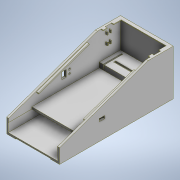
# Autodesk Inventor part: main
Saved by Autodesk Inventor 2021 (Build 250183000, 183)
## iProperties
Created: 2019-01-15
Part Number: main
Material: ABS 塑料(1)
Document SubType Name: Modeling
Designer: Guo Xin
Density: 1.06 g/cm^3
Appearance: 平滑 - 白色(1)
Author: Guo Xin
Autodesk Inventor part; units mm, degrees
note: some values were not read from the file. Chosen so that the rebuilt part matches the saved one: second side of "拉伸16".
ref_plane "YZ Plane" through (0, 0, 0) normal (1, 0, 0) x (0, 1, 0)
ref_plane "XZ Plane" through (0, 0, 0) normal (0, 1, 0) x (-1, 0, 0)
ref_plane "XY Plane" through (0, 0, 0) normal (0, 0, 1) x (1, 0, 0)
sketch "草图1" plane through (0, 0, 0) normal (0, 1, 0) x (-1, 0, 0)
  line L0 (0, 0) -> (80, 0)
  line L1 (80, 0) -> (80, -172)
  line L2 (80, -172) -> (0, -172)
  line L3 (0, -172) -> (0, 0)
  dimension "d0" = 172
  dimension "d1" = 80
  constraints: 8 end point, 2 parallel, 1 horizontal, 1 perpendicular
  measures "d0" distance between parallel lines of L2 L0
  measures "d1" distance between parallel lines of L3 L1
extrude "拉伸1" add sketch "草图1" along normal blind 70
sketch "草图2" plane through (-80, 0, 0) normal (0, 0, 1) x (1, 0, 0)
  line L0 (2.5, 16.5) -> (77.5, 16.5)
  line L1 (77.5, 16.5) -> (77.5, 3)
  line L2 (77.5, 3) -> (2.5, 3)
  line L3 (2.5, 3) -> (2.5, 16.5)
  line L4 (80, 0) -> (0, 0) projected
  line L5 (80, 0) -> (80, 70) projected
  line L6 (0, 0) -> (0, 70) projected
  dimension "d4" = 3
  dimension "d5" = 2.5
  dimension "d6" = 2.5
  dimension "d7" = 13.5
  dimension "d225" = 75
  constraints: 8 end point, 2 parallel, 1 horizontal, 1 perpendicular
  measures "d4" distance between parallel lines of L4 L2
  measures "d5" distance between parallel lines of L5 L1
  measures "d6" distance between parallel lines of L6 L3
  measures "d7" distance between parallel lines of L2 L0
  measures "d225" distance between parallel lines of L1 L3
extrude "拉伸2" cut sketch "草图2" against normal blind 170
sketch "草图3" plane through (0, 70, 0) normal (0, 1, 0) x (1, 0, 0)
  line L0 (-66.25, 151) -> (-13.75, 151)
  line L1 (-13.75, 151) -> (-13.75, 148)
  line L2 (-13.75, 148) -> (-66.25, 148)
  line L3 (-66.25, 148) -> (-66.25, 151)
  line L4 (0, 172) -> (-80, 172) projected
  line L5 (-80, 172) -> (-80, 0) projected
  line L6 (0, 0) -> (0, 172) projected
  dimension "d10" = 52.5
  dimension "d11" = 3
  dimension "d12" = 21
  dimension "d13" = 13.75
  dimension "d14" = 80
  constraints: 8 end point, 2 parallel, 1 horizontal, 1 perpendicular
  measures "d10" distance between parallel lines of L1 L3
  measures "d11" distance between parallel lines of L2 L0
  measures "d12" distance between parallel lines of L4 L0
  measures "d13" distance between parallel lines of L5 L3
  measures "d14" distance between parallel lines of L6 L5
extrude "拉伸3" cut sketch "草图3" against normal blind 45
sketch "草图4" plane through (0, 0, 0) normal (1, 0, 0) x (0, 0, -1)
  line L0 (137, 70) -> (0, 22)
  line L1 (172, 0) -> (172, 70) projected
  line L2 (172, 0) -> (0, 0) projected
  line L3 (0, 0) -> (0, 70) projected
  line L4 (0, 70) -> (172, 70) projected
  dimension "d17" = 35
  dimension "d18" = 22
  constraints: 2 end point, 2 point on line
  measures "d17" distance from line of L1 L0.start
  measures "d18" distance from line of L2 L0.end
extrude "拉伸4" cut sketch "草图4" against normal blind 80 contours L0 L3 L4
sketch "草图5" plane through (0, 70, 0) normal (0, 1, 0) x (1, 0, 0)
  line L0 (-77, 137) -> (-3, 137)
  line L1 (-3, 137) -> (-3, 0)
  line L2 (-3, 0) -> (-77, 0)
  line L3 (-77, 0) -> (-77, 137)
  line L4 (-80, 0) -> (-80, 137) projected
  line L5 (0, 137) -> (0, 0) projected
  line L6 (-80, 137) -> (0, 137) projected
  line L7 (0, 0) -> (-80, 0) projected
  point P0 (-76, 137)
  point P1 (-76, 0)
  dimension "d21" = 3
  dimension "d22" = 3
  constraints: 8 end point, 2 collinear, 2 parallel, 1 horizontal, 1 perpendicular
  measures "d21" distance between parallel lines of L4 L3
  measures "d22" distance between parallel lines of L5 L1
extrude "拉伸5" cut sketch "草图5" against normal blind 48 contours L0 L1 L2 L3
sketch "草图9" plane through (-77, 70, -137) normal (0, 0, 1) x (1, 0, 0)
  line L0 (3, -3) -> (71, -3)
  line L1 (71, -3) -> (71, -43)
  line L2 (71, -43) -> (3, -43)
  line L3 (3, -43) -> (3, -3)
  line L4 (0, 0) -> (74, 0) projected
  line L5 (0, -48) -> (0, 0) projected
  line L6 (74, 0) -> (74, -48) projected
  line L7 (2.5, -48) -> (71.5, -48) projected
  point P0 (77, -70)
  dimension "d34" = 3
  dimension "d35" = 3
  dimension "d36" = 3
  dimension "d226" = 40
  constraints: 8 end point, 2 parallel, 1 horizontal, 1 perpendicular
  measures "d34" distance between parallel lines of L4 L0
  measures "d35" distance between parallel lines of L5 L3
  measures "d36" distance between parallel lines of L6 L1
  measures "d226" distance between parallel lines of L2 L0
extrude "拉伸8" cut sketch "草图9" against normal blind 32
sketch "草图12" plane through (-74, 27, -137) normal (1, 0, 0) x (0, 0, -1)
  line L0 (11, 40) -> (14, 40)
  line L1 (14, 40) -> (14, 0)
  line L2 (14, 0) -> (11, 0)
  line L3 (11, 0) -> (11, 40)
  line L4 (11, 43) -> (11, 40) projected
  line L5 (14, 43) -> (14, 40) projected
  line L6 (11, 40) -> (14, 40) projected
  line L7 (0, 0) -> (32, 0) projected
  point P0 (-137, -27)
  point P1 (11, -2)
  point P2 (14, -2)
  dimension "d40" = 0
  dimension "d41" = 0
  constraints: 8 end point, 2 collinear, 2 parallel, 1 horizontal, 1 perpendicular
  measures "d40" distance between parallel lines of L4 L3
  measures "d41" distance between parallel lines of L5 L1
extrude "拉伸9" cut sketch "草图12" against normal blind 3 and the other way blind 71
sketch "草图15" plane through (-74, 27, -137) normal (1, 0, 0) x (0, 0, -1)
  line L0 (0, 40) -> (6.5, 40)
  line L1 (6.5, 40) -> (6.5, 0)
  line L2 (6.5, 0) -> (0, 0)
  line L3 (0, 0) -> (0, 40)
  line L4 (0, 0) -> (0, 40) projected
  line L5 (0, 0) -> (32, 0) projected
  line L6 (0, 40) -> (32, 40) projected
  line L7 (11, 0) -> (11, 40) projected
  point P0 (-137, -27)
  dimension "d44" = 4.5
  constraints: 8 end point, 3 collinear, 2 parallel, 1 horizontal, 1 perpendicular
  measures "d44" distance between parallel lines of L7 L1
extrude "拉伸10" cut sketch "草图15" against normal blind 3 and the other way blind 71 contours L0 L1 L2 L3
sketch "草图16" plane through (-74, 27, -169) normal (1, 0, 0) x (0, 0, -1)
  line L0 (-13.5, 40) -> (0, 40)
  line L1 (0, 40) -> (0, 0)
  line L2 (0, 0) -> (-13.5, 0)
  line L3 (-13.5, 0) -> (-13.5, 40)
  line L4 (-18, 0) -> (0, 0) projected
  line L5 (-18, 40) -> (0, 40) projected
  line L6 (-18, 40) -> (-18, 0) projected
  line L7 (0, 0) -> (0, 40) projected
  point P0 (-169, -27)
  dimension "d47" = 4.5
  constraints: 8 end point, 3 collinear, 2 parallel, 1 horizontal, 1 perpendicular
  measures "d47" distance between parallel lines of L6 L3
extrude "拉伸11" cut sketch "草图16" against normal blind 3 and the other way blind 71 contours L0 L1 L2 L3
sketch "草图17" plane through (-74, 27, -148) normal (1, 0, 0) x (0, 0, -1)
  line L0 (-0.75, 40) -> (3.75, 40)
  line L1 (3.75, 40) -> (3.75, 19)
  line L2 (3.75, 19) -> (-0.75, 19)
  line L3 (-0.75, 19) -> (-0.75, 40)
  line L4 (3, 40) -> (7.5, 40) projected
  line L5 (0, 0) -> (0, 40) projected
  line L6 (3, 0) -> (7.5, 0) projected
  point P0 (-148, -27)
  dimension "d50" = 0.75
  dimension "d51" = 4.5
  dimension "d52" = 19
  constraints: 8 end point, 2 parallel, 1 collinear, 1 horizontal, 1 perpendicular
  measures "d50" distance between parallel lines of L5 L3
  measures "d51" distance between parallel lines of L1 L3
  measures "d52" distance between parallel lines of L6 L2
extrude "拉伸12" cut sketch "草图17" against normal blind 3 and the other way blind 71
sketch "草图18" plane through (-74, 27, -143.5) normal (1, 0, 0) x (0, 0, -1)
  line L0 (0, 18) -> (12, 18)
  line L1 (12, 18) -> (12, 0)
  line L2 (12, 0) -> (0, 0)
  line L3 (0, 0) -> (0, 18)
  line L4 (0, 40) -> (0, 0) projected
  line L5 (12, 0) -> (12, 40) projected
  line L6 (7.5, 0) -> (12, 0) projected
  line L7 (8.25, 19) -> (3.75, 19) projected
  point P0 (-143.5, -27)
  point P1 (4.5, 19)
  dimension "d55" = 1
  constraints: 8 end point, 3 collinear, 2 parallel, 1 horizontal, 1 perpendicular
  measures "d55" distance between parallel lines of L0 L7
extrude "拉伸13" cut sketch "草图18" against normal blind 3 and the other way blind 71
sketch "草图19" plane through (-74, 46, -147.25) normal (1, 0, 0) x (0, 0, -1)
  line L0 (-3.75, 21) -> (-1, 21)
  line L1 (-1, 21) -> (-1, -1)
  line L2 (-1, -1) -> (-3.75, -1)
  line L3 (-3.75, -1) -> (-3.75, 21)
  line L4 (5.5, 21) -> (8.25, 21)
  line L5 (8.25, 21) -> (8.25, -1)
  line L6 (8.25, -1) -> (5.5, -1)
  line L7 (5.5, -1) -> (5.5, 21)
  line L8 (2.25, 24.0103) -> (2.25, -3.9452)
  line L9 (0, 0) -> (0, 21) projected
  line L10 (-3.75, 21) -> (0, 21) projected
  line L11 (-3.75, 21) -> (-3.75, -1) projected
  line L12 (-3.75, -1) -> (8.25, -1) projected
  point P0 (-147.25, -46)
  point P1 (0.75, -1)
  dimension "d58" = 2.25
  dimension "d59" = 2
  constraints: 18 end point, 4 parallel, 3 collinear, 2 horizontal, 2 perpendicular, 1 point on line, 1 vertical, 3 other
  measures "d58" distance between parallel lines of L8 L9
  measures "d59" diameter of L1 L9
extrude "拉伸14" cut sketch "草图19" against normal blind 3 and the other way blind 71
sketch "草图20" plane through (-74, 46, -147.25) normal (1, 0, 0) x (0, 0, -1)
  line L0 (-1, 13) -> (5.5, 13)
  line L1 (5.5, 13) -> (5.5, 3)
  line L2 (5.5, 3) -> (-1, 3)
  line L3 (-1, 3) -> (-1, 13)
  line L4 (-1, 21) -> (-1, -1) projected
  line L5 (5.5, -1) -> (5.5, 21) projected
  line L6 (-1, -1) -> (5.5, -1) projected
  line L7 (0.75, 21) -> (3.75, 21) projected
  line L8 (0, 13) -> (-1, 13)
  line L9 (0, 0) -> (0, 21) projected
  line L10 (-1, 21) -> (0, 21) projected
  point P0 (-147.25, -46)
  point P1 (0.75, -1)
  dimension "d62" = 4
  dimension "d63" = 8
  constraints: 10 end point, 3 collinear, 2 parallel, 1 horizontal, 1 perpendicular
  measures "d62" distance between parallel lines of L6 L2
  measures "d63" distance between parallel lines of L7 L0
extrude "拉伸15" cut sketch "草图20" against normal blind 3 and the other way blind 71 contours L0 L9 L2 L3 | L0 L1 L2 L9
sketch "草图21" plane through (0, 22, 0) normal (0, 1, 0) x (1, 0, 0)
  line L0 (-71.25, 165) -> (-69.5, 165)
  line L1 (-69.5, 165) -> (-69.5, 135)
  line L2 (-69.5, 135) -> (-71.25, 135)
  line L3 (-71.25, 135) -> (-71.25, 165)
  line L4 (-10.5, 165) -> (-8.75, 165)
  line L5 (-8.75, 165) -> (-8.75, 135)
  line L6 (-8.75, 135) -> (-10.5, 135)
  line L7 (-10.5, 135) -> (-10.5, 165)
  line L8 (-3, 135) -> (-77, 135) projected
  line L9 (-66.25, 148) -> (-66.25, 151) projected
  line L10 (-2.5, 170) -> (-77.5, 170) projected
  line L11 (-80, 0) -> (-80, 172) projected
  line L12 (-40, 178.7655) -> (-40, 86)
  point P0 (0, 0)
  dimension "d94" = 5
  dimension "d95" = 1.75
  dimension "d96" = 5
  dimension "d97" = 10.5
  dimension "d188" = 80
  constraints: 18 end point, 4 parallel, 2 horizontal, 2 perpendicular, 1 collinear, 1 point on line, 1 vertical, 3 other
  measures "d94" distance between parallel lines of L9 L3
  measures "d95" distance between parallel lines of L1 L3
  measures "d96" distance between parallel lines of L10 L0
  measures "d97" distance between parallel lines of L11 L1
  measures "d188" diameter of L11 L12
extrude "拉伸16" cut sketch "草图21" along normal blind 5
sketch "草图29" plane through (-74, 67, -146.25) normal (1, 0, 0) x (0, 0, -1)
  line L0 (0, 0) -> (6.5, 0)
  line L1 (6.5, 0) -> (6.5, -4)
  line L2 (6.5, -4) -> (0, -4)
  line L3 (0, -4) -> (0, 0)
  line L4 (0, 0) -> (1, 0) projected
  line L5 (0, 0) -> (0, -8) projected
  line L6 (6.5, -8) -> (6.5, 0) projected
  point P0 (-146.25, -67)
  dimension "d248" = 4
  constraints: 8 end point, 3 collinear, 2 parallel, 1 horizontal, 1 perpendicular
  measures "d248" distance between parallel lines of L2 L0
extrude "拉伸20" cut sketch "草图29" against normal blind 3 and the other way blind 65
sketch "草图30" plane through (-3, 27, -169) normal (-1, 0, 0) x (0, 0, 1)
  line L0 (32, 41.9404) -> (32, 39.8212)
  line L1 (32, 39.8212) -> (127.0364, 6.5238)
  line L2 (127.0364, 6.5238) -> (127.0364, 8.643)
  line L3 (127.0364, 8.643) -> (32, 41.9404)
  line L4 (32, 43) -> (32, 40) projected
  line L5 (32, 39.8212) -> (32.992, 42.6524)
  line L6 (32, 43) -> (169, -5) projected
  line L7 (127.0364, 8.643) -> (126.3751, 6.7555)
  line L8 (32, 39.8212) -> (126.3751, 6.7555)
  line L9 (126.3751, 6.7555) -> (126.7057, 7.6992)
  line L10 (126.7057, 7.6992) -> (32.3307, 40.7649)
  line L11 (32.3307, 40.7649) -> (32, 39.8212)
  point P0 (169, -27)
  point P1 (169, -5)
  point P2 (32, -5)
  point P3 (157.5833, 0)
  dimension "d144" = 1
  dimension "d145" = 2
  dimension "d146" = 100
  dimension "d147" = 2
  dimension "d148" = 1
  constraints: 20 end point, 3 collinear, 3 parallel, 3 perpendicular, 1 point on line, 1 vertical, 5 other
  measures "d145" distance between parallel lines of L1 L3
  measures "d146" distance between parallel lines of L7 L5
  measures "d147" distance between parallel lines of L3 L8
  measures "d148" distance between parallel lines of L1 L10
extrude "拉伸21" add sketch "草图30" along normal blind 74 contours L3 L5 L0 | L3 L7 L10 L5 | L5 L10 L7 L1
sketch "草图31" plane through (-77, 35.643, -41.9636) normal (0, 0.9437509, 0.3306573) x (1, 0, 0)
  line L0 (3, 101.0511) -> (71, 101.0511)
  line L1 (71, 101.0511) -> (71, 0)
  line L2 (71, 0) -> (3, 0)
  line L3 (3, 0) -> (3, 101.0511)
  line L4 (0, 101.0511) -> (74, 101.0511) projected
  line L5 (74, 0) -> (0, 0) projected
  line L6 (0, -44.1143) -> (0, 101.0511) projected
  line L7 (74, 101.0511) -> (74, -44.1143) projected
  point P0 (77, -51.3888)
  point P1 (4, 0)
  point P2 (0, -32.0172)
  point P3 (74, -32.0172)
  dimension "d151" = 3
  dimension "d152" = 3
  constraints: 8 end point, 2 collinear, 2 parallel, 1 horizontal, 1 perpendicular
  measures "d151" distance between parallel lines of L6 L3
  measures "d152" distance between parallel lines of L7 L1
extrude "拉伸22" cut sketch "草图31" against normal blind 2 contours L0 L1 L2 L3
sketch "草图36" plane through (0, 0, 0) normal (0, -1, 0) x (1, 0, 0)
  line L0 (-13.5, 0) -> (-66.5, 0)
  line L1 (-66.5, 0) -> (-66.5, -10)
  line L2 (-66.5, -10) -> (-13.5, -10)
  line L3 (-13.5, -10) -> (-13.5, 0)
  line L4 (-80, 0) -> (-80, -172) projected
  line L5 (0, -172) -> (0, 0) projected
  line L6 (0, 0) -> (-80, 0) projected
  dimension "d159" = 80
  dimension "d160" = 13.5
  dimension "d161" = 13.5
  dimension "d162" = 10
  constraints: 8 end point, 2 parallel, 1 collinear, 1 horizontal, 1 perpendicular
  measures "d159" distance between parallel lines of L4 L5
  measures "d160" distance between parallel lines of L3 L5
  measures "d161" distance between parallel lines of L4 L1
  measures "d162" distance between parallel lines of L0 L2
extrude "拉伸23" cut sketch "草图36" against normal blind 1
sketch "草图37" plane through (0, 1, 0) normal (0, -1, 0) x (1, 0, 0)
  line L0 (-13.5, 0) -> (-13.5, -10) projected
  line L1 (-66.5, -10) -> (-66.5, 0) projected
  line L2 (-13.5, -10) -> (-66.5, -10) projected
  point P0 (0, 0)
  point P1 (-21.5, -4)
  point P2 (-58.5, -4)
  dimension "d165" = 8
  dimension "d166" = 8
  dimension "d167" = 6
  dimension "d168" = 6
  measures "d165" distance from line of L0 point (-21.5, -4)
  measures "d166" distance from line of L1 point (-58.5, -4)
  measures "d167" distance from line of L2 point (-21.5, -4)
  measures "d168" distance from line of L2 point (-58.5, -4)
hole "孔1" at (-21.5, 1, -4) at (-58.5, 1, -4) direction (0, 1, 0) diameter 2.013 depth 1 tip angle 118 thread size "M2.5x0.45" class "6H" standard "ISO Metric profile"
sketch "草图41" plane through (-77, 27, -169) normal (1, 0, 0) x (0, 0, -1)
  line L0 (-88.681, 15.4425) -> (-82.181, 15.4425)
  line L1 (-82.181, 15.4425) -> (-82.181, 5.4425)
  line L2 (-82.181, 5.4425) -> (-88.681, 5.4425)
  line L3 (-88.681, 5.4425) -> (-88.681, 15.4425)
  circle A0 centre (-77.181, 13.4425) radius 1.5
  circle A1 centre (-77.181, 7.4425) radius 1.5
  line L4 (-169, -5) -> (0, -5) projected
  line L5 (-96.0528, 10.4425) -> (-76.3132, 10.4425)
  point P0 (-169, -27)
  point P1 (0, 0)
  point P2 (-157.5833, 0)
  dimension "d181" = 6.5
  dimension "d182" = 10
  dimension "d184" = 3
  dimension "d185" = 6
  dimension "d242" = 5
  constraints: 10 end point, 3 horizontal, 2 centre point, 2 parallel, 1 perpendicular, 1 symmetric about line, 2 other
  measures "d181" distance between parallel lines of L1 L3
  measures "d182" distance between parallel lines of L2 L0
  measures "d184" diameter of A0
  measures "d185" diameter of A0.centre L5
  measures "d242" distance from line of L1 A0.centre
extrude "拉伸24" cut sketch "草图41" against normal blind 10
sketch "草图42" plane through (0, 22, 0) normal (0, 1, 0) x (1, 0, 0)
  line L0 (-74.5, 0) -> (-77, 0)
  line L1 (-77, 0) -> (-77, 35)
  line L2 (-77, 35) -> (-74.5, 35)
  line L3 (-74.5, 35) -> (-74.5, 0)
  line L4 (-77, 0) -> (-77, 137) projected
  line L5 (-3, 0) -> (-77, 0) projected
  line L6 (-74.5, 0) -> (-74.5, 135) projected
  line L7 (-74.5, 35) -> (-5.5, 35) projected
  line L8 (-5.5, 0) -> (-3, 0)
  line L9 (-3, 0) -> (-3, 35)
  line L10 (-3, 35) -> (-5.5, 35)
  line L11 (-5.5, 35) -> (-5.5, 0)
  line L12 (-5.5, 135) -> (-5.5, 0) projected
  line L13 (-3, 137) -> (-3, 0) projected
  line L14 (-3, 0) -> (-77, 0) projected
  point P0 (0, 0)
  point P1 (-77, 11.4167)
  point P2 (-3, 11.4167)
  constraints: 16 end point, 8 collinear, 4 parallel, 2 horizontal, 2 perpendicular
extrude "拉伸25" cut sketch "草图42" against normal blind 10 contours L0 L1 L2 L3 | L11 L10 L9 L5
sketch "草图43" plane through (0, 22, 0) normal (0, 1, 0) x (1, 0, 0)
  line L0 (-66.25, 151) -> (-13.75, 151) projected
  line L1 (-66.25, 148) -> (-66.25, 151) projected
  line L2 (-13.75, 148) -> (-66.25, 148) projected
  line L3 (-13.75, 151) -> (-13.75, 148) projected
  line L4 (-77, 35) -> (-74.5, 35) projected
  line L5 (-71.25, 137) -> (-71.25, 165) projected
  line L6 (-69.5, 165) -> (-69.5, 137) projected
  line L7 (-10.5, 137) -> (-10.5, 165) projected
  line L8 (-8.75, 165) -> (-8.75, 137) projected
  line L9 (-5.5, 35) -> (-3, 35) projected
  line L10 (-77, 137) -> (-71.25, 137) projected
  line L11 (-8.75, 137) -> (-3, 137) projected
  line L12 (-69.5, 137) -> (-10.5, 137) projected
  line L13 (-10.5, 165) -> (-8.75, 165) projected
  line L14 (-71.25, 165) -> (-69.5, 165) projected
  line L15 (-3, 137) -> (-3, 35) projected
  line L16 (-77, 35) -> (-77, 137) projected
  line L17 (-74.5, 35) -> (-74.5, 0) projected
  line L18 (-5.5, 0) -> (-74.5, 0) projected
  line L19 (-5.5, 0) -> (-5.5, 35) projected
  point P0 (0, 0)
extrude "拉伸26" add sketch "草图43" along normal blind 4 contours L0 L3 L2 L1
sketch "草图48" plane through (-2.5, 3, -170) normal (-1, 0, 0) x (0, 0, 1)
  line L0 (52, 23) -> (69, 23)
  line L1 (69, 23) -> (69, 33.7)
  line L2 (69, 33.7) -> (52, 33.7)
  line L3 (52, 33.7) -> (52, 23)
  line L4 (1, 19) -> (135, 19) projected
  line L5 (35, 19) -> (35, 17.8) projected
  point P0 (170, -3)
  point P1 (1, 24)
  dimension "d208" = 17
  dimension "d209" = 10.7
  dimension "d210" = 4
  dimension "d211" = 17
  constraints: 8 end point, 2 parallel, 1 horizontal, 1 perpendicular, 1 other
  measures "d208" distance between parallel lines of L1 L3
  measures "d209" distance between parallel lines of L2 L0
  measures "d211" distance between parallel lines of L5 L3
extrude "拉伸29" cut sketch "草图48" against normal blind 3 and the other way blind 1
sketch "草图52" plane through (0, 70, 0) normal (0, 1, 0) x (1, 0, 0)
  line L0 (-80, 172) -> (0, 172)
  line L1 (0, 172) -> (0, 127)
  line L2 (0, 127) -> (-80, 127)
  line L3 (-80, 127) -> (-80, 172)
  line L4 (0, 172) -> (-80, 172) projected
  line L5 (-80, 172) -> (-80, 137) projected
  line L6 (-77, 137) -> (-3, 137) projected
  line L7 (0, 137) -> (0, 172) projected
  point P0 (0, 0)
  dimension "d258" = 45
  constraints: 8 end point, 3 collinear, 2 parallel, 1 horizontal, 1 perpendicular
  measures "d258" distance between parallel lines of L2 L0
extrude "拉伸30" cut sketch "草图52" against normal blind 1
sketch "草图53" plane through (-74, 68.9404, -137) normal (0, 0, 1) x (1, 0, 0)
  line L0 (0, 0.0596) -> (68, 0.0596)
  line L1 (68, 0.0596) -> (68, -1.9404)
  line L2 (68, -1.9404) -> (0, -1.9404)
  line L3 (0, -1.9404) -> (0, 0.0596)
  line L4 (71, 0.0596) -> (-3, 0.0596) projected
  line L5 (68, -1.9404) -> (0, -1.9404) projected
  line L6 (-3, 0.0596) -> (-3, 0) projected
  line L7 (68, 0.0596) -> (68, -1.7717) projected
  line L8 (71, 0.0596) -> (71, -46.9404) projected
  point P0 (74, -68.9404)
  point P1 (-3, -1.9404)
  point P2 (71, 1.0596)
  dimension "d237" = 3
  dimension "d241" = 3
  constraints: 8 end point, 2 collinear, 2 parallel, 1 horizontal, 1 perpendicular
  measures "d237" distance between parallel lines of L3 L6
  measures "d241" distance between parallel lines of L8 L1
extrude "拉伸31" cut sketch "草图53" against normal blind 32
sketch "草图54" plane through (0, 69, 0) normal (0, 1, 0) x (1, 0, 0)
  line L0 (-80, 172) -> (0, 172)
  line L1 (0, 172) -> (0, 137)
  line L2 (0, 137) -> (-80, 137)
  line L3 (-80, 137) -> (-80, 172)
  line L4 (-80, 172) -> (0, 172) projected
  line L5 (-80, 134.1458) -> (-80, 172) projected
  line L6 (-74, 137) -> (-77, 137) projected
  line L7 (0, 172) -> (0, 134.1458) projected
  line L8 (-40, 172) -> (-40, 135.8653)
  line L9 (-77, 155.75) -> (-74, 155.75)
  line L10 (-74, 155.75) -> (-74, 145.75)
  line L11 (-74, 145.75) -> (-77, 145.75)
  line L12 (-77, 145.75) -> (-77, 155.75)
  line L13 (-6, 155.75) -> (-3, 155.75)
  line L14 (-6, 145.75) -> (-3, 145.75)
  line L15 (-74, 137) -> (-74, 169) projected
  line L16 (-77, 137) -> (-77, 169) projected
  line L17 (-6, 155.75) -> (-3, 155.75)
  line L18 (-3, 155.75) -> (-3, 145.75)
  line L19 (-3, 145.75) -> (-6, 145.75)
  line L20 (-6, 145.75) -> (-6, 155.75)
  point P0 (0, 0)
  point P1 (-77, 147.25)
  point P2 (-74, 147.25)
  dimension "d255" = 10
  constraints: 28 end point, 6 collinear, 6 parallel, 5 perpendicular, 2 horizontal, 1 midpoint, 6 other
  measures "d255" distance between parallel lines of L11 L9
extrude "拉伸32" cut sketch "草图54" against normal blind 3 contours L12 L9 L10 L11 | L13 L18 L14 L20
sketch "草图55" plane through (-6, 35.643, -41.9636) normal (0, 0.9437509, 0.3306573) x (1, 0, 0)
  line L0 (-71, 100.7204) -> (-68, 100.7204)
  line L1 (-68, 100.7204) -> (-68, 80.7204)
  line L2 (-68, 80.7204) -> (-71, 80.7204)
  line L3 (-71, 80.7204) -> (-71, 100.7204)
  line L4 (0, 100.7204) -> (3, 100.7204)
  line L5 (3, 100.7204) -> (3, 80.7204)
  line L6 (3, 80.7204) -> (0, 80.7204)
  line L7 (0, 80.7204) -> (0, 100.7204)
  line L8 (3, 100.7204) -> (0, 100.7204) projected
  line L9 (0, 100.7007) -> (0, 0) projected
  line L10 (3, 98.0268) -> (3, -44.1143) projected
  line L11 (-71, -44.1143) -> (-71, 98.0268) projected
  line L12 (-68, 0) -> (-68, 100.7007) projected
  point P0 (6, -51.3888)
  point P1 (3, 101.0511)
  point P2 (-71, 101.0511)
  dimension "d245" = 20
  constraints: 16 end point, 5 collinear, 4 parallel, 2 horizontal, 2 perpendicular, 2 point on line
  measures "d245" distance between parallel lines of L2 L0
extrude "拉伸33" cut sketch "草图55" against normal blind 3
sketch "草图56" plane through (0, 69, 0) normal (0, 1, 0) x (1, 0, 0)
  line L0 (-77, 137) -> (-3, 137)
  line L1 (-3, 137) -> (-3, 140)
  line L2 (-3, 140) -> (-77, 140)
  line L3 (-77, 140) -> (-77, 137)
  line L4 (-74, 137) -> (-77, 137) projected
  line L5 (-77, 137.7007) -> (-77, 145.75) projected
  line L6 (-3, 145.75) -> (-3, 137.7007) projected
  point P0 (0, 0)
  point P1 (-3, 146.25)
  dimension "d249" = 3
  constraints: 8 end point, 3 collinear, 2 parallel, 1 horizontal, 1 perpendicular
  measures "d249" distance between parallel lines of L0 L2
extrude "拉伸34" cut sketch "草图56" against normal blind 3
sketch "草图57" plane through (-77, 69, -140) normal (0, 0, 1) x (1, 0, 0)
  line L0 (0, -1) -> (74, -1)
  line L1 (74, -1) -> (74, -2)
  line L2 (74, -2) -> (0, -2)
  line L3 (0, -2) -> (0, -1)
  line L4 (3, -2) -> (0, -2) projected
  line L5 (0, -47) -> (0, 0) projected
  line L6 (74, 0) -> (74, -47) projected
  point P0 (77, -69)
  point P1 (0, 1)
  point P2 (74, 1)
  dimension "d252" = 1
  constraints: 8 end point, 3 collinear, 2 parallel, 1 horizontal, 1 perpendicular
  measures "d252" distance between parallel lines of L2 L0
extrude "拉伸35" cut sketch "草图57" against normal blind 29
sketch "草图58" plane through (-77, 70, -169) normal (0, 0, 1) x (1, 0, 0)
  line L0 (3, -1) -> (71, -1)
  line L1 (71, -1) -> (71, -2)
  line L2 (71, -2) -> (3, -2)
  line L3 (3, -2) -> (3, -1)
  line L4 (3, -1) -> (71, -1) projected
  line L5 (0, -2) -> (3, -2) projected
  line L6 (3, -1) -> (3, -2) projected
  line L7 (71, -2) -> (71, -1) projected
  point P0 (77, -70)
  constraints: 8 end point, 4 collinear, 2 parallel, 1 horizontal, 1 perpendicular
extrude "拉伸36" add sketch "草图58" along normal blind 2
sketch "草图61" plane through (0, 22, 0) normal (0, 1, 0) x (1, 0, 0)
  line L0 (-74.5, 35) -> (-5.5, 35)
  line L1 (-5.5, 35) -> (-5.5, 0)
  line L2 (-5.5, 0) -> (-74.5, 0)
  line L3 (-74.5, 0) -> (-74.5, 35)
  line L4 (-77, 35) -> (-74.5, 35) projected
  line L5 (-74.5, 35) -> (-74.5, 0) projected
  line L6 (-5.5, 0) -> (-74.5, 0) projected
  line L7 (-5.5, 0) -> (-5.5, 35) projected
  point P0 (0, 0)
  constraints: 8 end point, 4 collinear, 2 parallel, 1 horizontal, 1 perpendicular
extrude "拉伸38" cut sketch "草图61" against normal blind 10
sketch "草图62" plane through (-3, 16.5, 0) normal (-1, 0, 0) x (0, 0, 1)
  line L0 (-68, 13.5) -> (-60, 13.5)
  line L1 (-60, 13.5) -> (-60, 9.5)
  line L2 (-60, 9.5) -> (-68, 9.5)
  line L3 (-68, 9.5) -> (-68, 13.5)
  line L4 (-137, 5.5) -> (-35, 5.5) projected
  line L5 (-35, 5.5) -> (-35, 0) projected
  point P0 (0, -16.5)
  dimension "d282" = 8
  dimension "d283" = 4
  dimension "d284" = 4
  dimension "d285" = 25
  constraints: 8 end point, 2 parallel, 1 horizontal, 1 perpendicular
  measures "d282" distance between parallel lines of L1 L3
  measures "d283" distance between parallel lines of L2 L4
  measures "d284" distance between parallel lines of L2 L0
  measures "d285" distance between parallel lines of L5 L1
extrude "拉伸39" cut sketch "草图62" against normal blind 10
sketch "草图67" plane through (-77, 22, -35) normal (0, 0, 1) x (1, 0, 0)
  line L0 (0, 0) -> (74, 0)
  line L1 (74, 0) -> (74, -2.5)
  line L2 (74, -2.5) -> (0, -2.5)
  line L3 (0, -2.5) -> (0, 0)
  line L4 (0, 0) -> (74, 0) projected
  line L5 (74, 0) -> (74, -5.5) projected
  line L6 (0, -5.5) -> (0, 0) projected
  line L7 (74, -5.5) -> (0, -5.5) projected
  point P0 (77, -22)
  dimension "d292" = 3
  constraints: 8 end point, 3 collinear, 2 parallel, 1 horizontal, 1 perpendicular
  measures "d292" distance between parallel lines of L7 L2
extrude "拉伸40" cut sketch "草图67" against normal blind 102 contours L0 L1 L2 L3
sketch "草图68" plane through (0, 26, 0) normal (0, 1, 0) x (1, 0, 0)
  line L0 (-66.25, 151) -> (-13.75, 151)
  line L1 (-13.75, 151) -> (-13.75, 148)
  line L2 (-13.75, 148) -> (-66.25, 148)
  line L3 (-66.25, 148) -> (-66.25, 151)
  line L4 (-13.75, 151) -> (-66.25, 151) projected
  line L5 (-66.25, 151) -> (-66.25, 148) projected
  line L6 (-66.25, 148) -> (-13.75, 148) projected
  line L7 (-13.75, 148) -> (-13.75, 151) projected
  point P0 (0, 0)
  constraints: 8 end point, 4 collinear, 2 parallel, 1 horizontal, 1 perpendicular
extrude "拉伸41" cut sketch "草图68" against normal blind 1
sketch "草图69" plane through (0, 0, 0) normal (1, 0, 0) x (0, 0, -1)
  line L0 (101, 36.7) -> (101, 26) projected
  line L1 (101, 26) -> (118, 26) projected
  line L2 (101, 36.7) -> (118, 36.7)
  line L3 (118, 36.7) -> (118, 26)
  line L4 (118, 26) -> (101, 26)
  line L5 (101, 26) -> (101, 36.7)
  point P0 (0, 0)
  constraints: 8 end point, 2 parallel, 1 horizontal, 1 perpendicular
extrude "拉伸42" add sketch "草图69" against normal blind 1
